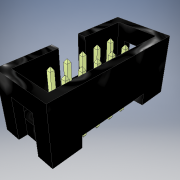
# Autodesk Inventor part: PinHeader-2x5-Male
Saved by Autodesk Inventor 2018 (Build 220112000, 112)
## iProperties
Created: 2020-04-18
Part Number: PinHeader-2x5-Male
Material: Všeobecné
Document SubType Name: Modeling
Designer: Jozko Mrkvicka
Density: 1 g/cm^3
Appearance: Výchozí
Author: Jozko Mrkvicka
Autodesk Inventor part; units mm, degrees
ref_plane "YZ Plane" through (0, 0, 0) normal (1, 0, 0) x (0, 1, 0)
ref_plane "XZ Plane" through (0, 0, 0) normal (0, 1, 0) x (-1, 0, 0)
ref_plane "XY Plane" through (0, 0, 0) normal (0, 0, 1) x (1, 0, 0)
sketch "Náčrt1" plane through (0, 0, 0) normal (0, 1, 0) x (-1, 0, 0)
  line L0 (0, 0) -> (8.89, 0)
  line L1 (8.89, 0) -> (8.89, -20.32)
  line L2 (8.89, -20.32) -> (0, -20.32)
  line L3 (0, -20.32) -> (0, 0)
  dimension "d0" = 8.89
  dimension "d1" = 20.32
  constraints: 8 end point, 2 parallel, 1 horizontal, 1 perpendicular
  measures "d0" distance of L1.end L2.end
  measures "d1" distance of L0.end L1.end
extrude "Vysunutí1" add sketch "Náčrt1" along normal blind 2.54
sketch "Náčrt2" plane through (0, 2.54, 0) normal (0, 1, 0) x (1, 0, 0)
  line L0 (-1.27, 1.2688) -> (-7.5834, 1.2688)
  line L1 (-7.5834, 19.05) -> (-1.27, 19.05)
  line L2 (-1.27, 19.05) -> (-1.27, 1.2688)
  line L3 (-8.89, 7.9375) -> (-7.5834, 7.9375)
  line L4 (-7.5834, 12.3825) -> (-8.89, 12.3825)
  line L5 (-7.5834, 1.2688) -> (-7.5834, 7.9375)
  line L6 (-7.5834, 12.3825) -> (-7.5834, 19.05)
  line L7 (-8.89, 20.32) -> (0, 20.32) projected
  line L8 (0, 0) -> (-8.89, 0)
  line L9 (-8.89, 20.32) -> (0, 20.32)
  line L10 (0, 20.32) -> (0, 0)
  line L11 (-8.89, 0) -> (-8.89, 7.9375)
  line L12 (-8.89, 12.3825) -> (-8.89, 20.32)
  point P0 (-7.62, 10.16)
  point P1 (-7.62, 10.16)
  point P2 (-7.62, 10.16)
  dimension "d9" = 4.445
  constraints: 24 end point, 7 parallel, 4 perpendicular, 3 horizontal, 2 point on line, 1 vertical
  measures "d9" distance between parallel lines of L4 L3
extrude "Vysunutí2" add sketch "Náčrt2" along normal blind 6.35
sketch "Náčrt3" plane through (0, 0, 0) normal (0, -1, 0) x (1, 0, 0)
  line L0 (-6.35, 0) -> (-6.35, -1.27)
  line L1 (-6.35, -1.27) -> (-2.54, -1.27)
  line L2 (-2.54, -1.27) -> (-2.54, 0)
  line L3 (-2.54, 0) -> (-6.35, 0)
  line L4 (-6.35, 0) -> (-6.35, -1.27)
  line L5 (-6.35, -20.32) -> (-6.35, -19.05)
  line L6 (-6.35, -19.05) -> (-2.54, -19.05)
  line L7 (-2.54, -19.05) -> (-2.54, -20.32)
  line L8 (-2.54, -20.32) -> (-6.35, -20.32)
  line L9 (-6.35, -20.32) -> (-6.35, -19.05)
  constraints: 20 end point, 2 parallel, 1 horizontal, 1 perpendicular
extrude "Vysunutí3" cut sketch "Náčrt3" against normal blind 6.35
sketch "Náčrt4" plane through (0, 2.54, 0) normal (0, 1, 0) x (1, 0, 0)
  line L0 (-8.89, 0) -> (-8.89, 20.32) projected
  line L1 (0, 20.32) -> (0, 0) projected
  line L2 (-6.0325, 4.7625) -> (-5.3975, 4.7625)
  line L3 (-5.3975, 4.7625) -> (-5.3975, 5.3975)
  line L4 (-5.3975, 5.3975) -> (-6.0325, 5.3975)
  line L5 (-6.0325, 5.3975) -> (-6.0325, 4.7625)
  line L6 (-6.0325, 7.3025) -> (-5.3975, 7.3025)
  line L7 (-5.3975, 7.3025) -> (-5.3975, 7.9375)
  line L8 (-5.3975, 7.9375) -> (-6.0325, 7.9375)
  line L9 (-6.0325, 7.9375) -> (-6.0325, 7.3025)
  line L10 (-3.4925, 4.7625) -> (-2.8575, 4.7625)
  line L11 (-2.8575, 4.7625) -> (-2.8575, 5.3975)
  line L12 (-2.8575, 5.3975) -> (-3.4925, 5.3975)
  line L13 (-3.4925, 5.3975) -> (-3.4925, 4.7625)
  line L14 (-3.4925, 7.3025) -> (-2.8575, 7.3025)
  line L15 (-2.8575, 7.3025) -> (-2.8575, 7.9375)
  line L16 (-2.8575, 7.9375) -> (-3.4925, 7.9375)
  line L17 (-3.4925, 7.9375) -> (-3.4925, 7.3025)
  line L18 (-3.4925, 9.8425) -> (-2.8575, 9.8425)
  line L19 (-2.8575, 9.8425) -> (-2.8575, 10.4775)
  line L20 (-2.8575, 10.4775) -> (-3.4925, 10.4775)
  line L21 (-3.4925, 10.4775) -> (-3.4925, 9.8425)
  line L22 (-6.0325, 9.8425) -> (-5.3975, 9.8425)
  line L23 (-5.3975, 9.8425) -> (-5.3975, 10.4775)
  line L24 (-5.3975, 10.4775) -> (-6.0325, 10.4775)
  line L25 (-6.0325, 10.4775) -> (-6.0325, 9.8425)
  line L26 (-6.0325, 12.3825) -> (-5.3975, 12.3825)
  line L27 (-5.3975, 12.3825) -> (-5.3975, 13.0175)
  line L28 (-5.3975, 13.0175) -> (-6.0325, 13.0175)
  line L29 (-6.0325, 13.0175) -> (-6.0325, 12.3825)
  line L30 (-6.0325, 14.9225) -> (-5.3975, 14.9225)
  line L31 (-5.3975, 14.9225) -> (-5.3975, 15.5575)
  line L32 (-5.3975, 15.5575) -> (-6.0325, 15.5575)
  line L33 (-6.0325, 15.5575) -> (-6.0325, 14.9225)
  line L34 (-3.4925, 12.3825) -> (-2.8575, 12.3825)
  line L35 (-2.8575, 12.3825) -> (-2.8575, 13.0175)
  line L36 (-2.8575, 13.0175) -> (-3.4925, 13.0175)
  line L37 (-3.4925, 13.0175) -> (-3.4925, 12.3825)
  line L38 (-3.4925, 14.9225) -> (-2.8575, 14.9225)
  line L39 (-2.8575, 14.9225) -> (-2.8575, 15.5575)
  line L40 (-2.8575, 15.5575) -> (-3.4925, 15.5575)
  line L41 (-3.4925, 15.5575) -> (-3.4925, 14.9225)
  constraints: 80 end point, 20 parallel, 10 horizontal, 10 perpendicular
extrude "Vysunutí4" add sketch "Náčrt4" along normal blind 5.715
sketch "Náčrt6" plane through (0, 0, 0) normal (0, -1, 0) x (1, 0, 0)
  line L0 (-1.905, -15.875) -> (0, -15.875)
  line L1 (-1.905, -4.445) -> (0, -4.445)
  line L2 (-1.905, -15.875) -> (0, -15.875)
  line L3 (0, -15.875) -> (0, -4.445)
  line L4 (0, -4.445) -> (-1.905, -4.445)
  line L5 (-1.905, -4.445) -> (-1.905, -15.875)
  point P0 (0, 0)
  point P1 (0, -20.32)
  constraints: 12 end point, 2 parallel, 1 horizontal, 1 perpendicular
extrude "Vysunutí6" cut sketch "Náčrt6" against normal blind 1.905
draft "PlochaZešikmení1" angle 45 pull direction (1, 0, 0) faces at (-1.27, 1.905, -8.255) fixed edges at (0, 1.905, -10.16)
sketch "Náčrt8" plane through (0, 0, 0) normal (0, -1, 0) x (1, 0, 0)
  line L0 (-3.4925, -12.3825) -> (-3.4925, -13.0175) projected
  line L1 (-3.4925, -13.0175) -> (-2.8575, -13.0175) projected
  line L2 (-2.8575, -13.0175) -> (-2.8575, -12.3825) projected
  line L3 (-2.8575, -12.3825) -> (-3.4925, -12.3825) projected
  line L4 (-6.0325, -12.3825) -> (-6.0325, -13.0175) projected
  line L5 (-6.0325, -13.0175) -> (-5.3975, -13.0175) projected
  line L6 (-5.3975, -13.0175) -> (-5.3975, -12.3825) projected
  line L7 (-5.3975, -12.3825) -> (-6.0325, -12.3825) projected
  line L8 (-3.4925, -9.8425) -> (-3.4925, -10.4775) projected
  line L9 (-3.4925, -10.4775) -> (-2.8575, -10.4775) projected
  line L10 (-2.8575, -10.4775) -> (-2.8575, -9.8425) projected
  line L11 (-2.8575, -9.8425) -> (-3.4925, -9.8425) projected
  line L12 (-3.4925, -4.7625) -> (-3.4925, -5.3975) projected
  line L13 (-3.4925, -5.3975) -> (-2.8575, -5.3975) projected
  line L14 (-2.8575, -5.3975) -> (-2.8575, -4.7625) projected
  line L15 (-2.8575, -4.7625) -> (-3.4925, -4.7625) projected
  line L16 (-6.0325, -4.7625) -> (-6.0325, -5.3975) projected
  line L17 (-6.0325, -5.3975) -> (-5.3975, -5.3975) projected
  line L18 (-5.3975, -5.3975) -> (-5.3975, -4.7625) projected
  line L19 (-5.3975, -4.7625) -> (-6.0325, -4.7625) projected
  line L20 (-6.0325, -7.3025) -> (-6.0325, -7.9375) projected
  line L21 (-6.0325, -7.9375) -> (-5.3975, -7.9375) projected
  line L22 (-5.3975, -7.9375) -> (-5.3975, -7.3025) projected
  line L23 (-5.3975, -7.3025) -> (-6.0325, -7.3025) projected
  line L24 (-2.8575, -7.9375) -> (-2.8575, -7.3025) projected
  line L25 (-2.8575, -7.3025) -> (-3.4925, -7.3025) projected
  line L26 (-3.4925, -7.3025) -> (-3.4925, -7.9375) projected
  line L27 (-3.4925, -7.9375) -> (-2.8575, -7.9375) projected
  line L28 (-6.0325, -9.8425) -> (-6.0325, -10.4775) projected
  line L29 (-6.0325, -10.4775) -> (-5.3975, -10.4775) projected
  line L30 (-5.3975, -10.4775) -> (-5.3975, -9.8425) projected
  line L31 (-5.3975, -9.8425) -> (-6.0325, -9.8425) projected
  line L32 (-3.4925, -14.9225) -> (-3.4925, -15.5575) projected
  line L33 (-3.4925, -15.5575) -> (-2.8575, -15.5575) projected
  line L34 (-2.8575, -15.5575) -> (-2.8575, -14.9225) projected
  line L35 (-2.8575, -14.9225) -> (-3.4925, -14.9225) projected
  line L36 (-6.0325, -14.9225) -> (-6.0325, -15.5575) projected
  line L37 (-6.0325, -15.5575) -> (-5.3975, -15.5575) projected
  line L38 (-5.3975, -15.5575) -> (-5.3975, -14.9225) projected
  line L39 (-5.3975, -14.9225) -> (-6.0325, -14.9225) projected
  line L40 (-2.54, -1.27) -> (-2.54, -1.2688) projected
  line L41 (-2.54, -1.2688) -> (-1.27, -1.2688) projected
  line L42 (-1.27, -1.2688) -> (-1.27, -19.05) projected
  line L43 (-1.27, -19.05) -> (-2.54, -19.05) projected
  line L44 (-2.54, -19.05) -> (-6.35, -19.05) projected
  line L45 (-6.35, -19.05) -> (-7.5834, -19.05) projected
  line L46 (-7.5834, -19.05) -> (-7.5834, -12.3825) projected
  line L47 (-7.5834, -12.3825) -> (-8.89, -12.3825) projected
  line L48 (-8.89, -12.3825) -> (-8.89, -7.9375) projected
  line L49 (-8.89, -7.9375) -> (-7.5834, -7.9375) projected
  line L50 (-7.5834, -7.9375) -> (-7.5834, -1.2688) projected
  line L51 (-7.5834, -1.2688) -> (-6.35, -1.2688) projected
  line L52 (-6.35, -1.2688) -> (-6.35, -1.27) projected
  line L53 (-6.35, -1.27) -> (-2.54, -1.27) projected
  point P0 (0, 0)
extrude "Vysunutí7" add sketch "Náčrt8" along normal blind 2.54 contours L3 L2 L1 L0 | L7 L6 L5 L4 | L11 L10 L9 L8 | L15 L14 L13 L12 | L19 L18 L17 L16 | L23 L22 L21 L20 | L27 L26 L25 L24 | L31 L30 L29 L28 | L35 L34 L33 L32 | L39 L38 L37 L36
chamfer "Zkosení21" distance 0.254 angle 60 4 edges at (-6.0325, -2.54, -15.24) (-5.715, -2.54, -15.5575) (-5.3975, -2.54, -15.24) (-5.715, -2.54, -14.9225) measured on face at (-5.9325, -2.54, -15.24) measured on face at (-5.715, -2.54, -15.0225) measured on face at (-5.4975, -2.54, -15.24) measured on face at (-5.715, -2.54, -15.4575)
chamfer "Zkosení22" distance 0.254 angle 60 4 edges at (-3.4925, -2.54, -15.24) (-3.175, -2.54, -15.5575) (-3.175, -2.54, -14.9225) (-2.8575, -2.54, -15.24) measured on face at (-2.9575, -2.54, -15.24) measured on face at (-3.175, -2.54, -15.4575) measured on face at (-3.3925, -2.54, -15.24) measured on face at (-3.175, -2.54, -15.0225)
chamfer "Zkosení23" distance 0.254 angle 60 4 edges at (-3.4925, -2.54, -12.7) (-3.175, -2.54, -13.0175) (-2.8575, -2.54, -12.7) (-3.175, -2.54, -12.3825) measured on face at (-3.175, -2.54, -12.4825) measured on face at (-2.9575, -2.54, -12.7) measured on face at (-3.175, -2.54, -12.9175) measured on face at (-3.3925, -2.54, -12.7)
chamfer "Zkosení24" distance 0.254 angle 60 4 edges at (-6.0325, -2.54, -12.7) (-5.715, -2.54, -13.0175) (-5.715, -2.54, -12.3825) (-5.3975, -2.54, -12.7) measured on face at (-5.4975, -2.54, -12.7) measured on face at (-5.9325, -2.54, -12.7) measured on face at (-5.715, -2.54, -12.4825) measured on face at (-5.715, -2.54, -12.9175)
chamfer "Zkosení25" distance 0.254 angle 60 4 edges at (-3.4925, -2.54, -10.16) (-3.175, -2.54, -10.4775) (-3.175, -2.54, -9.8425) (-2.8575, -2.54, -10.16) measured on face at (-3.175, -2.54, -9.9425) measured on face at (-2.9575, -2.54, -10.16) measured on face at (-3.175, -2.54, -10.3775) measured on face at (-3.3925, -2.54, -10.16)
chamfer "Zkosení26" distance 0.254 angle 60 4 edges at (-6.0325, -2.54, -10.16) (-5.715, -2.54, -10.4775) (-5.715, -2.54, -9.8425) (-5.3975, -2.54, -10.16) measured on face at (-5.9325, -2.54, -10.16) measured on face at (-5.4975, -2.54, -10.16) measured on face at (-5.715, -2.54, -9.9425) measured on face at (-5.715, -2.54, -10.3775)
chamfer "Zkosení27" distance 0.254 angle 60 4 edges at (-6.0325, -2.54, -7.62) (-5.715, -2.54, -7.9375) (-5.715, -2.54, -7.3025) (-5.3975, -2.54, -7.62) measured on face at (-5.715, -2.54, -7.8375) measured on face at (-5.9325, -2.54, -7.62) measured on face at (-5.715, -2.54, -7.4025) measured on face at (-5.4975, -2.54, -7.62)
chamfer "Zkosení28" distance 0.254 angle 60 4 edges at (-3.4925, -2.54, -7.62) (-3.175, -2.54, -7.9375) (-2.8575, -2.54, -7.62) (-3.175, -2.54, -7.3025) measured on face at (-2.9575, -2.54, -7.62) measured on face at (-3.175, -2.54, -7.4025) measured on face at (-3.175, -2.54, -7.8375) measured on face at (-3.3925, -2.54, -7.62)
chamfer "Zkosení29" distance 0.254 angle 60 4 edges at (-3.4925, -2.54, -5.08) (-3.175, -2.54, -5.3975) (-2.8575, -2.54, -5.08) (-3.175, -2.54, -4.7625) measured on face at (-2.9575, -2.54, -5.08) measured on face at (-3.175, -2.54, -4.8625) measured on face at (-3.175, -2.54, -5.2975) measured on face at (-3.3925, -2.54, -5.08)
chamfer "Zkosení30" distance 0.254 angle 60 4 edges at (-5.715, -2.54, -5.3975) (-6.0325, -2.54, -5.08) (-5.715, -2.54, -4.7625) (-5.3975, -2.54, -5.08) measured on face at (-5.4975, -2.54, -5.08) measured on face at (-5.9325, -2.54, -5.08) measured on face at (-5.715, -2.54, -4.8625) measured on face at (-5.715, -2.54, -5.2975)
chamfer "Zkosení31" distance 0.254 angle 60 4 edges at (-6.0325, 8.255, -5.08) (-5.715, 8.255, -4.7625) (-5.715, 8.255, -5.3975) (-5.3975, 8.255, -5.08) measured on face at (-5.715, 8.255, -4.8625) measured on face at (-5.715, 8.255, -5.2975) measured on face at (-5.4975, 8.255, -5.08) measured on face at (-5.9325, 8.255, -5.08)
chamfer "Zkosení32" distance 0.254 angle 60 4 edges at (-3.4925, 8.255, -5.08) (-3.175, 8.255, -4.7625) (-3.175, 8.255, -5.3975) (-2.8575, 8.255, -5.08) measured on face at (-3.175, 8.255, -5.2975) measured on face at (-3.3925, 8.255, -5.08) measured on face at (-3.175, 8.255, -4.8625) measured on face at (-2.9575, 8.255, -5.08)
chamfer "Zkosení33" distance 0.254 angle 60 4 edges at (-3.4925, 8.255, -7.62) (-3.175, 8.255, -7.3025) (-3.175, 8.255, -7.9375) (-2.8575, 8.255, -7.62) measured on face at (-3.175, 8.255, -7.8375) measured on face at (-3.3925, 8.255, -7.62) measured on face at (-3.175, 8.255, -7.4025) measured on face at (-2.9575, 8.255, -7.62)
chamfer "Zkosení34" distance 0.254 angle 60 4 edges at (-6.0325, 8.255, -7.62) (-5.715, 8.255, -7.3025) (-5.715, 8.255, -7.9375) (-5.3975, 8.255, -7.62) measured on face at (-5.715, 8.255, -7.8375) measured on face at (-5.4975, 8.255, -7.62) measured on face at (-5.9325, 8.255, -7.62) measured on face at (-5.715, 8.255, -7.4025)
chamfer "Zkosení35" distance 0.254 angle 60 4 edges at (-3.4925, 8.255, -10.16) (-3.175, 8.255, -9.8425) (-3.175, 8.255, -10.4775) (-2.8575, 8.255, -10.16) measured on face at (-3.175, 8.255, -10.3775) measured on face at (-3.3925, 8.255, -10.16) measured on face at (-3.175, 8.255, -9.9425) measured on face at (-2.9575, 8.255, -10.16)
chamfer "Zkosení36" distance 0.254 angle 60 4 edges at (-6.0325, 8.255, -10.16) (-5.715, 8.255, -10.4775) (-5.3975, 8.255, -10.16) (-5.715, 8.255, -9.8425) measured on face at (-5.715, 8.255, -10.3775) measured on face at (-5.4975, 8.255, -10.16) measured on face at (-5.9325, 8.255, -10.16) measured on face at (-5.715, 8.255, -9.9425)
chamfer "Zkosení37" distance 0.254 angle 60 4 edges at (-3.4925, 8.255, -12.7) (-3.175, 8.255, -13.0175) (-2.8575, 8.255, -12.7) (-3.175, 8.255, -12.3825) measured on face at (-3.175, 8.255, -12.9175) measured on face at (-2.9575, 8.255, -12.7) measured on face at (-3.3925, 8.255, -12.7) measured on face at (-3.175, 8.255, -12.4825)
chamfer "Zkosení38" distance 0.254 angle 60 4 edges at (-6.0325, 8.255, -12.7) (-5.715, 8.255, -13.0175) (-5.3975, 8.255, -12.7) (-5.715, 8.255, -12.3825) measured on face at (-5.715, 8.255, -12.9175) measured on face at (-5.4975, 8.255, -12.7) measured on face at (-5.9325, 8.255, -12.7) measured on face at (-5.715, 8.255, -12.4825)
chamfer "Zkosení39" distance 0.254 angle 60 4 edges at (-3.4925, 8.255, -15.24) (-3.175, 8.255, -15.5575) (-2.8575, 8.255, -15.24) (-3.175, 8.255, -14.9225) measured on face at (-3.175, 8.255, -15.4575) measured on face at (-3.3925, 8.255, -15.24) measured on face at (-2.9575, 8.255, -15.24) measured on face at (-3.175, 8.255, -15.0225)
chamfer "Zkosení40" distance 0.254 angle 60 4 edges at (-6.0325, 8.255, -15.24) (-5.715, 8.255, -15.5575) (-5.3975, 8.255, -15.24) (-5.715, 8.255, -14.9225) measured on face at (-5.4975, 8.255, -15.24) measured on face at (-5.715, 8.255, -15.4575) measured on face at (-5.9325, 8.255, -15.24) measured on face at (-5.715, 8.255, -15.0225)
